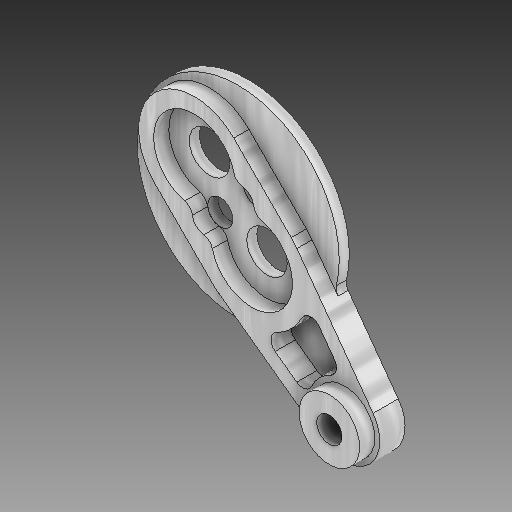
# Autodesk Inventor part: 脚クランク涙型1
Saved by Autodesk Inventor 2020 (Build 240168000, 168)
## iProperties
Created: 2019-07-23
Part Number: 脚クランク涙型1
Material: アルミニウム 7075
Document SubType Name: Modeling
Designer: 雪村
Density: 2.81 g/cm^3
Appearance: サテン - ブラシ仕上げ 重厚
Mass: 1.63241 g
Surface Area: 10.983 cm^2
Volume: 0.580927 cm^3
Description: アルミ7000 4t
Author: 雪村
Autodesk Inventor part; units mm, degrees
ref_plane "YZ Plane" through (0, 0, 0) normal (1, 0, 0) x (0, 1, 0)
ref_plane "XZ Plane" through (0, 0, 0) normal (0, 1, 0) x (-1, 0, 0)
ref_plane "XY Plane" through (0, 0, 0) normal (0, 0, 1) x (1, 0, 0)
sketch "スケッチ1" plane through (0, 0, 0) normal (0, 0, 1) x (1, 0, 0)
  line L0 (0, 0) -> (-12.0208, 12.0208)
  circle A0 centre (-9.1747, 9.1747) radius 2
  circle A1 centre (-14.8669, 14.8669) radius 2
  circle A2 centre (-14.8669, 14.8669) radius 4.025 construction
  circle A3 centre (-9.1747, 9.1747) radius 4.025 construction
  circle A4 centre (-13.7886, 10.253) radius 1.25
  circle A5 centre (-10.253, 13.7886) radius 1.25
  line L1 (-13.7886, 10.253) -> (-10.253, 13.7886) construction
  circle A6 centre (0, 0) radius 1.25
  arc A7 (-2.4749, 2.4749) -> (-2.0583, -2.8308) centre (0, 0) ccw construction
  arc A8 (-14.6971, 9.3445) -> (-9.5747, 16.4536) centre (-14.8669, 14.8669) ccw construction
  arc A9 (-14.467, 7.588) -> (-12.4239, 4.7061) centre (-9.1747, 9.1747) ccw
  line L2 (-12.4239, 4.7061) -> (-2.0583, -2.8308)
  line L3 (-4.7061, 12.4239) -> (2.8308, 2.0583)
  arc A10 (-11.1417, 16.3911) -> (-7.588, 14.467) centre (-10.253, 13.7886) ccw construction
  arc A11 (-16.4536, 9.5747) -> (-14.467, 7.588) centre (-13.7886, 10.253) ccw
  arc A12 (-16.3911, 11.1417) -> (-16.4536, 9.5747) centre (-13.7886, 10.253) ccw construction
  arc A13 (-14.467, 7.588) -> (-16.3911, 11.1417) centre (-13.7886, 10.253) ccw construction
  arc A14 (-16.4536, 9.5747) -> (-14.6971, 9.3445) centre (-14.8669, 14.8669) ccw construction
  arc A15 (-14.6971, 9.3445) -> (-14.467, 7.588) centre (-9.1747, 9.1747) ccw construction
  arc A16 (-9.5747, 16.4536) -> (-11.1417, 16.3911) centre (-10.253, 13.7886) ccw construction
  arc A17 (-7.588, 14.467) -> (-9.3445, 14.6971) centre (-9.1747, 9.1747) ccw construction
  arc A18 (-7.588, 14.467) -> (-9.5747, 16.4536) centre (-10.253, 13.7886) ccw
  arc A19 (-9.5747, 16.4536) -> (-16.4536, 9.5747) centre (-14.8669, 14.8669) ccw
  arc A20 (-9.3445, 14.6971) -> (-14.6971, 9.3445) centre (-9.1747, 9.1747) ccw construction
  arc A21 (-4.7061, 12.4239) -> (-7.588, 14.467) centre (-9.1747, 9.1747) ccw
  arc A22 (-12.4239, 4.7061) -> (-4.7061, 12.4239) centre (-9.1747, 9.1747) ccw construction
  arc A23 (2.8308, 2.0583) -> (-2.4749, 2.4749) centre (0, 0) ccw construction
  arc A24 (-2.0583, -2.8308) -> (2.8308, 2.0583) centre (0, 0) ccw
  circle A25 centre (-12.0208, 12.0208) radius 10
  point P0 (-2.4084, 9.2638)
  point P1 (-9.2638, 2.4084)
  dimension "d3" = 8.05
  dimension "d0" = 4
  dimension "d1" = 4
  dimension "d2" = 8.05
  dimension "d4" = 2.5
  dimension "d5" = 2.5
  dimension "d6" = 5
  dimension "d7" = 2.5
  dimension "d8" = 7
  dimension "d9" = 1.5
  dimension "d10" = 1.5
  dimension "d11" = 1.5
  dimension "d12" = 1.5
  dimension "d13" = 17
  dimension "d59" = 20
  constraints: 43 point on circle, 25 centre point, 12 tangent, 8 end point, 6 coincident, 3 point on line, 1 midpoint, 1 perpendicular, 4 other
  measures "d0" diameter of A0
  measures "d1" diameter of A1
  measures "d2" diameter of A2
  measures "d4" diameter of A4
  measures "d5" diameter of A5
  measures "d6" distance of L1.start L1.end
  measures "d7" diameter of A6
  measures "d8" diameter of A7
  measures "d9" radial gap between concentric circles of A2 A8
  measures "d11" radial gap between concentric circles of A5 A10
  measures "d12" radial gap between concentric circles of A4 A11
  measures "d13" distance of L0.start L0.end
  measures "d59" diameter of A25
extrude "押し出し1" add sketch "スケッチ1" along normal blind 4
sketch "スケッチ2" plane through (0, 0, 4) normal (0, 0, 1) x (1, 0, 0)
  circle A0 centre (-14.8669, 14.8669) radius 2 projected
  circle A1 centre (-13.7886, 10.253) radius 1.25 projected
  circle A2 centre (-10.253, 13.7886) radius 1.25 projected
  circle A3 centre (-9.1747, 9.1747) radius 2 projected
  circle A4 centre (-14.8669, 14.8669) radius 4.025
  circle A5 centre (-9.1747, 9.1747) radius 4.025
  point P0 (0, 0)
  point P1 (-10.842, 14.8911)
  point P2 (-14.8911, 10.842)
  point P3 (-13.0613, 11.2697)
  point P4 (-12.0208, 12.0208)
  point P5 (-11.2697, 13.0613)
  point P6 (-9.1505, 13.1996)
  point P7 (-10.9804, 12.772)
  point P8 (-12.772, 10.9804)
  point P9 (-13.1996, 9.1505)
  dimension "d17" = 8.05
  dimension "d18" = 8.05
  constraints: 2 centre point, 2 coincident
  measures "d17" diameter of A4
  measures "d18" diameter of A5
extrude "押し出し2" cut sketch "スケッチ2" against normal blind 3 contours A1 A5 A2 | A1 A4 A2
sketch "スケッチ3" plane through (0, 0, 4) normal (0, 0, 1) x (1, 0, 0)
  arc A0 (-13.0613, 11.2697) -> (-12.0208, 12.0208) centre (-14.8669, 14.8669) ccw projected
  arc A1 (-12.772, 10.9804) -> (-13.0613, 11.2697) centre (-13.7886, 10.253) ccw projected
  arc A2 (-12.0208, 12.0208) -> (-12.772, 10.9804) centre (-9.1747, 9.1747) ccw projected
  arc A3 (-12.0208, 12.0208) -> (-11.2697, 13.0613) centre (-14.8669, 14.8669) ccw projected
  arc A4 (-10.9804, 12.772) -> (-12.0208, 12.0208) centre (-9.1747, 9.1747) ccw projected
  arc A5 (-11.2697, 13.0613) -> (-10.9804, 12.772) centre (-10.253, 13.7886) ccw projected
  arc A6 (-13.0613, 11.2697) -> (-14.8911, 10.842) centre (-13.7886, 10.253) ccw projected
  circle A7 centre (-13.7886, 10.253) radius 1.275
  circle A8 centre (-10.253, 13.7886) radius 1.275
  point P0 (0, 0)
  point P1 (-11.2824, 13.0362)
  point P2 (-11.0055, 12.7593)
  point P3 (-13.0362, 11.2824)
  point P4 (-12.7593, 11.0055)
  dimension "d21" = 2.55
  dimension "d22" = 2.55
  constraints: 2 centre point, 2 coincident
  measures "d21" diameter of A7
  measures "d22" diameter of A8
extrude "押し出し3" cut sketch "スケッチ3" against normal blind 3
fillet "フィレット1" radius 1 4 edges at (-9.1224, 13.1994, 2.5) (-10.8423, 14.9193, 2.5) (-14.9193, 10.8423, 2.5) (-13.1994, 9.1224, 2.5)
sketch "スケッチ4" plane through (0, 0, 4) normal (0, 0, 1) x (1, 0, 0)
  circle A0 centre (0, 0) radius 1.25 projected
  circle A1 centre (0, 0) radius 3
  circle A2 centre (0, 0) radius 1.25 projected
  line L0 (-9.2638, 2.4084) -> (-2.0583, -2.8308) projected
  arc A3 (-2.0583, -2.8308) -> (2.8308, 2.0583) centre (0, 0) ccw projected
  line L1 (2.8308, 2.0583) -> (-2.4084, 9.2638) projected
  arc A4 (-2.4084, 9.2638) -> (-9.2638, 2.4084) centre (-12.0208, 12.0208) ccw projected
  arc A5 (-13.0871, 8.2291) -> (-13.9402, 8.9871) centre (-14.0591, 7.9942) ccw projected
  arc A6 (-15.0545, 10.1015) -> (-13.9402, 8.9871) centre (-13.7886, 10.253) ccw projected
  arc A7 (-15.0545, 10.1015) -> (-15.8125, 10.9546) centre (-16.0474, 9.9826) ccw projected
  arc A8 (-10.9546, 15.8125) -> (-15.8125, 10.9546) centre (-14.8669, 14.8669) ccw projected
  arc A9 (-10.9546, 15.8125) -> (-10.1015, 15.0545) centre (-9.9826, 16.0474) ccw projected
  arc A10 (-8.9871, 13.9402) -> (-10.1015, 15.0545) centre (-10.253, 13.7886) ccw projected
  arc A11 (-8.9871, 13.9402) -> (-8.2291, 13.0871) centre (-7.9942, 14.0591) ccw projected
  arc A12 (-13.0871, 8.2291) -> (-8.2291, 13.0871) centre (-9.1747, 9.1747) ccw projected
  dimension "d27" = 6
  constraints: 1 centre point, 1 coincident
  measures "d27" diameter of A1
extrude "押し出し4" cut sketch "スケッチ4" against normal blind 1.5 contours A4 L1 A3 L0
sketch "スケッチ8" plane through (0, 0, 2.5) normal (0, 0, 1) x (1, 0, 0)
  circle A0 centre (-9.1747, 9.1747) radius 2 projected
  circle A1 centre (-14.8669, 14.8669) radius 2 projected
  arc A2 (-10.9546, 15.8125) -> (-15.8125, 10.9546) centre (-14.8669, 14.8669) ccw projected
  circle A3 centre (-13.7886, 10.253) radius 1.25 projected
  arc A4 (-13.0871, 8.2291) -> (-8.2291, 13.0871) centre (-9.1747, 9.1747) ccw projected
  circle A5 centre (-10.253, 13.7886) radius 1.25 projected
  arc A6 (-8.9871, 13.9402) -> (-8.2291, 13.0871) centre (-7.9942, 14.0591) ccw projected
  arc A7 (-8.9871, 13.9402) -> (-10.1015, 15.0545) centre (-10.253, 13.7886) ccw projected
  arc A8 (-10.9546, 15.8125) -> (-10.1015, 15.0545) centre (-9.9826, 16.0474) ccw projected
  arc A9 (-15.0545, 10.1015) -> (-15.8125, 10.9546) centre (-16.0474, 9.9826) ccw projected
  arc A10 (-15.0545, 10.1015) -> (-13.9402, 8.9871) centre (-13.7886, 10.253) ccw projected
  arc A11 (-13.0871, 8.2291) -> (-13.9402, 8.9871) centre (-14.0591, 7.9942) ccw projected
  arc A12 (-9.5831, 16.4815) -> (-16.4815, 9.5831) centre (-14.8669, 14.8669) ccw
  arc A13 (-7.5601, 14.4585) -> (-9.5831, 16.4815) centre (-10.253, 13.7886) ccw
  arc A14 (-14.4585, 7.5601) -> (-7.5601, 14.4585) centre (-9.1747, 9.1747) ccw
  arc A15 (-16.4815, 9.5831) -> (-14.4585, 7.5601) centre (-13.7886, 10.253) ccw
  line L0 (-18.7737, 10.9602) -> (-13.0815, 5.2679)
  line L1 (-10.9602, 18.7737) -> (-5.2679, 13.0815)
  line L2 (-2.0583, -2.8308) -> (-9.2638, 2.4084) projected
  arc A16 (-2.4084, 9.2638) -> (-9.2638, 2.4084) centre (-12.0208, 12.0208) ccw projected
  line L3 (-2.0583, -2.8308) -> (-9.2638, 2.4084) projected
  arc A17 (-2.0583, -2.8308) -> (2.8308, 2.0583) centre (0, 0) ccw projected
  line L4 (-2.4084, 9.2638) -> (2.8308, 2.0583) projected
  circle A18 centre (0, 0) radius 3 projected
  arc A19 (-10.9546, 15.8125) -> (-15.8125, 10.9546) centre (-14.8669, 14.8669) ccw projected
  arc A20 (-10.9546, 15.8125) -> (-10.1015, 15.0545) centre (-9.9826, 16.0474) ccw projected
  arc A21 (-8.9871, 13.9402) -> (-10.1015, 15.0545) centre (-10.253, 13.7886) ccw projected
  arc A22 (-8.9871, 13.9402) -> (-8.2291, 13.0871) centre (-7.9942, 14.0591) ccw projected
  arc A23 (-13.0871, 8.2291) -> (-8.2291, 13.0871) centre (-9.1747, 9.1747) ccw projected
  arc A24 (-13.0871, 8.2291) -> (-13.9402, 8.9871) centre (-14.0591, 7.9942) ccw projected
  arc A25 (-15.0545, 10.1015) -> (-13.9402, 8.9871) centre (-13.7886, 10.253) ccw projected
  arc A26 (-15.0545, 10.1015) -> (-15.8125, 10.9546) centre (-16.0474, 9.9826) ccw projected
  line L5 (-12.4239, 4.7061) -> (-9.2638, 2.4084)
  line L6 (-4.7061, 12.4239) -> (-2.4084, 9.2638)
  dimension "d61" = 1.5
  constraints: 14 point on circle, 8 end point, 6 tangent, 4 centre point, 3 other
  measures "d61" radial gap between concentric circles of A2 A12
extrude "押し出し8" cut sketch "スケッチ8" against normal blind 1.5 contours A12 L0 A14 L5 A16 L6 L1
sketch "スケッチ9" plane through (0, 0, 2.5) normal (0, 0, 1) x (1, 0, 0)
  circle A0 centre (-9.1747, 9.1747) radius 2 projected
  circle A1 centre (-14.8669, 14.8669) radius 2 projected
  circle A2 centre (0, 0) radius 3 projected
  circle A3 centre (0, 0) radius 3.5
  arc A4 (-14.4585, 7.5601) -> (-7.5601, 14.4585) centre (-9.1747, 9.1747) ccw
  arc A5 (-16.4815, 9.5831) -> (-14.4585, 7.5601) centre (-13.7886, 10.253) ccw
  arc A6 (-9.5831, 16.4815) -> (-16.4815, 9.5831) centre (-14.8669, 14.8669) ccw
  arc A7 (-7.5601, 14.4585) -> (-9.5831, 16.4815) centre (-10.253, 13.7886) ccw
  line L0 (-2.4084, 9.2638) -> (2.8308, 2.0583) projected
  line L1 (-2.0583, -2.8308) -> (-9.2638, 2.4084) projected
  line L2 (-3.9623, 8.8502) -> (1.6176, 1.1762)
  line L3 (-1.1762, -1.6176) -> (-8.8502, 3.9623)
  arc A8 (-10.9546, 15.8125) -> (-15.8125, 10.9546) centre (-14.8669, 14.8669) ccw projected
  circle A9 centre (-13.7886, 10.253) radius 1.25 projected
  arc A10 (-13.0871, 8.2291) -> (-8.2291, 13.0871) centre (-9.1747, 9.1747) ccw projected
  circle A11 centre (-10.253, 13.7886) radius 1.25 projected
  arc A12 (-8.9871, 13.9402) -> (-8.2291, 13.0871) centre (-7.9942, 14.0591) ccw projected
  arc A13 (-8.9871, 13.9402) -> (-10.1015, 15.0545) centre (-10.253, 13.7886) ccw projected
  arc A14 (-10.9546, 15.8125) -> (-10.1015, 15.0545) centre (-9.9826, 16.0474) ccw projected
  arc A15 (-15.0545, 10.1015) -> (-15.8125, 10.9546) centre (-16.0474, 9.9826) ccw projected
  arc A16 (-15.0545, 10.1015) -> (-13.9402, 8.9871) centre (-13.7886, 10.253) ccw projected
  arc A17 (-13.0871, 8.2291) -> (-13.9402, 8.9871) centre (-14.0591, 7.9942) ccw projected
  point P0 (-8.4806, 3.6935)
  point P1 (-3.4993, 0.0715)
  point P2 (-0.0715, 3.4993)
  point P3 (-3.6935, 8.4806)
  dimension "d48" = 0.5
  dimension "d50" = 1.5
  dimension "d51" = 1.5
  constraints: 8 point on circle, 5 centre point, 4 end point, 2 parallel
  measures "d48" radial gap between concentric circles of A2 A3
  measures "d50" distance between parallel lines of L0 L2
  measures "d51" distance between parallel lines of L1 L3
extrude "押し出し9" cut sketch "スケッチ9" against normal through all contours A3 L3 A4 L2
fillet "フィレット4" radius 1 4 edges at (-8.4806, 3.6935, 1.25) (-3.4993, 0.0715, 1.25) (-3.6935, 8.4806, 1.25) (-0.0715, 3.4993, 1.25)
fillet "フィレット6" radius 1 2 edges at (-9.2638, 2.4084, 0.5) (-2.4084, 9.2638, 0.5)
sketch "スケッチ10" plane through (0, 0, 0) normal (0, 0, -1) x (-1, 0, 0)
  line L0 (0.9626, 4.7248) -> (2.5193, 6.8657) projected
  arc A0 (4.2241, 6.7216) -> (2.5193, 6.8657) centre (3.3281, 6.2776) ccw projected
  arc A1 (4.2241, 6.7216) -> (6.7216, 4.2241) centre (9.1747, 9.1747) ccw projected
  arc A2 (6.8657, 2.5193) -> (6.7216, 4.2241) centre (6.2776, 3.3281) ccw projected
  line L1 (6.8657, 2.5193) -> (4.7248, 0.9626) projected
  arc A3 (3.2174, 1.3778) -> (4.7248, 0.9626) centre (4.1367, 1.7714) ccw projected
  arc A4 (3.2174, 1.3778) -> (1.3778, 3.2174) centre (0, 0) ccw projected
  arc A5 (0.9626, 4.7248) -> (1.3778, 3.2174) centre (1.7714, 4.1367) ccw projected
  line L2 (-2.8308, 2.0583) -> (2.1298, 8.8806) projected
  arc A6 (-2.8308, 2.0583) -> (2.0583, -2.8308) centre (0, 0) ccw projected
  line L3 (8.8806, 2.1298) -> (2.0583, -2.8308) projected
  arc A7 (9.7007, 2.2937) -> (8.8806, 2.1298) centre (9.4687, 1.321) ccw projected
  arc A8 (9.7007, 2.2937) -> (2.2937, 9.7007) centre (12.0208, 12.0208) ccw projected
  arc A9 (2.1298, 8.8806) -> (2.2937, 9.7007) centre (1.321, 9.4687) ccw projected
  circle A10 centre (9.1747, 9.1747) radius 2 projected
  circle A11 centre (0, 0) radius 1.25 projected
  circle A12 centre (14.8669, 14.8669) radius 2 projected
  circle A13 centre (10.253, 13.7886) radius 1.25 projected
  circle A14 centre (13.7886, 10.253) radius 1.25 projected
extrude "押し出し10" add sketch "スケッチ10" against normal blind 0.5 contours L0 A0 A1 A2 L1 A3 A4 A5
sketch "スケッチ11" plane through (0, 0, 4) normal (0, 0, 1) x (1, 0, 0)
  circle A0 centre (0, 0) radius 3 projected
  arc A1 (-10.9546, 15.8125) -> (-15.8125, 10.9546) centre (-14.8669, 14.8669) ccw projected
  arc A2 (-10.9546, 15.8125) -> (-10.1015, 15.0545) centre (-9.9826, 16.0474) ccw projected
  arc A3 (-8.9871, 13.9402) -> (-10.1015, 15.0545) centre (-10.253, 13.7886) ccw projected
  arc A4 (-8.9871, 13.9402) -> (-8.2291, 13.0871) centre (-7.9942, 14.0591) ccw projected
  arc A5 (-13.0871, 8.2291) -> (-8.2291, 13.0871) centre (-9.1747, 9.1747) ccw projected
  arc A6 (-13.0871, 8.2291) -> (-13.9402, 8.9871) centre (-14.0591, 7.9942) ccw projected
  arc A7 (-15.0545, 10.1015) -> (-13.9402, 8.9871) centre (-13.7886, 10.253) ccw projected
  arc A8 (-15.0545, 10.1015) -> (-15.8125, 10.9546) centre (-16.0474, 9.9826) ccw projected
  arc A9 (-1.3778, 3.2174) -> (-3.2174, 1.3778) centre (0, 0) ccw projected
  arc A10 (-1.3778, 3.2174) -> (-0.9626, 4.7248) centre (-1.7714, 4.1367) ccw projected
  line L0 (-2.5193, 6.8657) -> (-0.9626, 4.7248) projected
  arc A11 (-2.5193, 6.8657) -> (-4.2241, 6.7216) centre (-3.3281, 6.2776) ccw projected
  arc A12 (-6.7216, 4.2241) -> (-4.2241, 6.7216) centre (-9.1747, 9.1747) ccw projected
  arc A13 (-6.7216, 4.2241) -> (-6.8657, 2.5193) centre (-6.2776, 3.3281) ccw projected
  line L1 (-4.7248, 0.9626) -> (-6.8657, 2.5193) projected
  arc A14 (-4.7248, 0.9626) -> (-3.2174, 1.3778) centre (-4.1367, 1.7714) ccw projected
  line L2 (2.8308, 2.0583) -> (-4.7061, 12.4239) projected
  line L3 (-5.2679, 13.0815) -> (-10.9602, 18.7737) projected
  arc A15 (-10.9602, 18.7737) -> (-18.7737, 10.9602) centre (-14.8669, 14.8669) ccw projected
  line L4 (-18.7737, 10.9602) -> (-13.0815, 5.2679) projected
  arc A16 (-13.0815, 5.2679) -> (-12.4239, 4.7061) centre (-9.1747, 9.1747) ccw projected
  line L5 (-2.0583, -2.8308) -> (-12.4239, 4.7061) projected
  arc A17 (-4.7061, 12.4239) -> (-5.2679, 13.0815) centre (-9.1747, 9.1747) ccw projected
  arc A18 (-2.0583, -2.8308) -> (2.8308, 2.0583) centre (0, 0) ccw projected
  line L6 (2.8308, 2.0583) -> (-2.1298, 8.8806) projected
  arc A19 (-2.0583, -2.8308) -> (2.8308, 2.0583) centre (0, 0) ccw projected
  line L7 (-8.8806, 2.1298) -> (-2.0583, -2.8308) projected
  arc A20 (-8.8806, 2.1298) -> (-9.7007, 2.2937) centre (-9.4687, 1.321) ccw projected
  arc A21 (-2.2937, 9.7007) -> (-9.7007, 2.2937) centre (-12.0208, 12.0208) ccw projected
  arc A22 (-2.2937, 9.7007) -> (-2.1298, 8.8806) centre (-1.321, 9.4687) ccw projected
  circle A23 centre (-9.1747, 9.1747) radius 2 projected
  circle A24 centre (0, 0) radius 1.25 projected
  circle A25 centre (-14.8669, 14.8669) radius 2 projected
  circle A26 centre (-10.253, 13.7886) radius 1.25 projected
  circle A27 centre (-13.7886, 10.253) radius 1.25 projected
equation "\"d3\" = d2"
equation "\"d0\" = d1"
equation "\"d21\" = d22"
